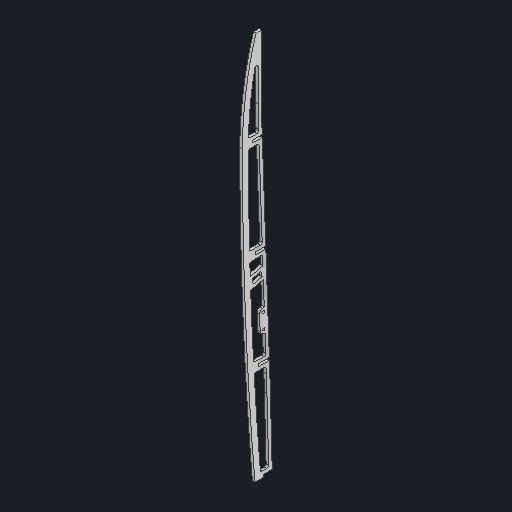
# Autodesk Inventor part: stringer_cowl
Saved by Autodesk Inventor 2023 (Build 270158030, 158C)
## iProperties
Created: 2022-03-23
Part Number: stringer_cowl
Material: Generic
Document SubType Name: Modeling
Designer: kardo
Density: 1 g/cm^3
Appearance: Default
Mass: 17.0204 g
Surface Area: 170.958 cm^2
Volume: 17.0204 cm^3
Author: kardo
Autodesk Inventor part; units mm, degrees
ref_plane "YZ Plane" through (0, 0, 0) normal (1, 0, 0) x (0, 1, 0)
ref_plane "XZ Plane" through (0, 0, 0) normal (0, 1, 0) x (-1, 0, 0)
ref_plane "XY Plane" through (0, 0, 0) normal (0, 0, 1) x (1, 0, 0)
derived "parameters_frame.ipt"
derived "surface_body.ipt"
sketch "sk_rail_top_cowl" plane through (54.6, 0, 0) normal (1, 0, 0) x (0, 1, 0)
  spline S0 degree 2 poles (-345, 39.712) (-172.656, 54.3934) (0, 54.4) knots 0 0 0 1 1 1
  spline S1 degree 3 poles (0, 54.4) (37.026, 54.4) (80.784, 47.9917) (112.2, 37.536) knots 1 1 1 1 2 2 2 2
  point P0 (0, 0)
sketch "sk_rail_bottom_standoff" plane through (34.32, 0, 0) normal (1, 0, 0) x (0, 1, 0)
  line L0 (-345, 16.32) -> (-262.2001, 18.586)
  arc A0 (-262.2001, 18.586) -> (-241.5001, 19.2432) centre (-326.8578, 2381.2399) ccw
  line L1 (36.465, 28.832) -> (112.2, 28.832)
  arc A1 (36.465, 28.832) -> (11.22, 28.376) centre (36.465, -670.197) ccw
  line L2 (-241.5001, 19.2432) -> (11.22, 28.376)
  line L3 (-465, 0) -> (375, 0) construction
  line L4 (11.22, 28.376) -> (11.22, 0) construction
  line L5 (-241.5001, 19.2432) -> (-241.5001, 0) construction
  point P0 (0, 0)
  point P1 (-241.5001, 19.1524)
  point P2 (11.22, 28.832)
ref_plane "plane_middle" through (0, 0, 0) normal (0, 1, 0) x (-1, 0, 0)
ref_plane "plane_rear" through (0, -345, 0) normal (0, 1, 0) x (-1, 0, 0)
ref_plane "plane_cowl_right" through (54.6, 0, 0) normal (1, 0, 0) x (0, 1, 0)
ref_plane "plane_nose" through (0, 112.2, 0) normal (0, 1, 0) x (-1, 0, 0)
ref_plane "plane_tail_1" through (0, -114.9999, 0) normal (0, 1, 0) x (-1, 0, 0)
ref_plane "plane_tail_2" through (0, -230.0001, 0) normal (0, 1, 0) x (-1, 0, 0)
derived "stencil_frame.ipt"
sketch "sk_cowl_joint_locations" plane through (54.6, 0, 0) normal (1, 0, 0) x (0, 1, 0)
  line L0 (-345, 16.32) -> (-262.2001, 18.586) construction
  arc A0 (-262.2001, 18.586) -> (-241.5001, 19.2432) centre (-326.8578, 2381.2399) ccw construction
  line L1 (-241.5001, 19.2432) -> (11.22, 28.376) construction
  arc A1 (36.465, 28.832) -> (11.22, 28.376) centre (36.465, -670.197) ccw construction
  line L2 (36.465, 28.832) -> (112.2, 28.832) construction
  line L3 (94.8, 29.632) -> (36.465, 29.632) construction
  arc A2 (36.465, 29.632) -> (11.1911, 29.1755) centre (36.465, -670.197) ccw construction
  line L4 (11.1911, 29.1755) -> (-241.529, 20.0427) construction
  arc A3 (-262.222, 19.3857) -> (-241.529, 20.0427) centre (-326.8578, 2381.2399) ccw construction
  line L5 (-262.222, 19.3857) -> (-345, 17.1203) construction
  line L6 (-230.0001, 3089.1136) -> (-230.0001, -1866.0023) construction
  line L7 (-114.9999, 3089.1136) -> (-114.9999, -1866.0023) construction
  line L8 (-345, 3089.1136) -> (-345, -1866.0023) construction
  line L9 (0, 3089.1136) -> (0, -1866.0023) construction
  line L10 (-230.0001, 44.8681) -> (-230.0001, 20.4593) construction
  line L11 (-114.9999, 49.7658) -> (-114.9999, 24.6152) construction
  line L12 (-345, 17.1203) -> (-345, 17.1203)
  line L13 (-345, 17.1203) -> (-345, 36.7228) construction
  line L14 (-850.7464, 3011.9134) -> (325.2296, -1886.3794) construction
  line L15 (-344.7454, 36.7228) -> (-345, 39.712) construction
  spline S0 degree 2 poles (-345, 39.712) (-172.656, 54.3934) (0, 54.4) knots 0 0 0 1 1 1
  spline S1 degree 3 poles (0, 54.4) (37.026, 54.4) (80.784, 47.9917) (112.2, 37.536) knots 1 1 1 1 2 2 2 2
  line L16 (0, 51.4) -> (0, 28.7711) construction
  spline S2 degree 3 poles (111.2526, 34.6895) (106.0906, 36.4075) (96.4401, 39.2282) (84.5011, 42.0313) (75.2591, 43.9395) (68.9709, 45.1125) (60.9945, 46.449) (54.5373, 47.4124) (46.413, 48.4791) (39.8882, 49.2203) (31.7426, 50.0013) (25.2514, 50.5076) (17.2112, 50.9875) (9.2661, 51.3118) (3.0567, 51.4) (0, 51.4) knots 1 1 1 1 1.166667 1.291667 1.333333 1.416667 1.458333 1.541667 1.583333 1.666667 1.708333 1.791667 1.833333 1.916667 2 2 2 2
  spline S3 degree 3 poles (0, 51.4) (-19.1698, 51.3993) (-52.712, 51.1604) (-91.0357, 50.4121) (-119.7742, 49.6473) (-138.931, 49.0355) (-162.8744, 48.1436) (-182.0269, 47.3282) (-205.9648, 46.1816) (-225.113, 45.1626) (-249.0455, 43.7615) (-268.1894, 42.5387) (-292.1166, 40.883) (-316.041, 39.1) (-335.1777, 37.5379) (-344.7454, 36.7228) knots 0 0 0 0 0.166667 0.291667 0.333333 0.416667 0.458333 0.541666 0.583333 0.666666 0.708333 0.791666 0.833333 0.916666 1 1 1 1
  line L17 (-144.5331, 44.6212) -> (-139.5174, 23.7292) construction
  line L18 (-134.9371, 30.3529) -> (-140.7713, 28.9522) construction
  line L19 (-137.4449, 40.7989) -> (-143.2792, 39.3982) construction
  line L20 (-144.5331, 44.6212) -> (-138.6989, 46.0219) construction
  line L21 (-139.5174, 23.7292) -> (-133.6831, 25.1299) construction
  line L22 (-138.6989, 46.0219) -> (-138.9044, 52.0184) construction
  point P0 (0, 0)
  point P1 (-345, 26.9216)
  point P2 (-230.0001, 32.6637)
  point P3 (-114.9999, 37.1905)
  point P4 (0, 40.0855)
  point P5 (-850.7464, 3011.9134)
  point P6 (325.2296, -1886.3794)
  point P7 (-85.2629, 50.788)
  point P8 (0, 40.0855)
sketch "sk_servo_mount" plane through (-54.6, 0, 0) normal (1, 0, 0) x (0, 1, 0)
  line L0 (-241.5001, 19.2432) -> (11.22, 28.376) construction
  line L1 (-345, 3089.1136) -> (-345, -1866.0023) construction
  line L2 (0, 3089.1136) -> (0, -1866.0023) construction
  line L3 (-195.0702, 20.9211) -> (-195.2941, 27.117) construction
  line L4 (-195.2941, 27.117) -> (-177.3059, 27.7671) construction
  line L5 (-177.3059, 27.7671) -> (-177.082, 21.5711) construction
  point P0 (0, 0)
  point P1 (-186.3, 27.4421)
sketch "sk_base" plane through (54.6, 0, 0) normal (1, 0, 0) x (0, 1, 0)
  line L0 (-345, 16.32) -> (-262.2001, 18.586) construction
  arc A0 (-262.2001, 18.586) -> (-241.5001, 19.2432) centre (-326.8578, 2381.2399) ccw construction
  line L1 (-241.5001, 19.2432) -> (11.22, 28.376) construction
  arc A1 (36.465, 28.832) -> (11.22, 28.376) centre (36.465, -670.197) ccw construction
  line L2 (36.465, 28.832) -> (112.2, 28.832) construction
  spline S0 degree 3 poles (0, 54.4) (37.026, 54.4) (80.784, 47.9917) (112.2, 37.536) knots 1 1 1 1 2 2 2 2 construction
  spline S1 degree 2 poles (-345, 39.712) (-172.656, 54.3934) (0, 54.4) knots 0 0 0 1 1 1 construction
  line L3 (-345, 2991.5273) -> (-345, -1280.4843) projected
  line L4 (112.2, 2991.5273) -> (112.2, -1280.4843) construction
  line L5 (109.2, 29.632) -> (36.465, 29.632)
  arc A2 (36.465, 29.632) -> (11.1911, 29.1755) centre (36.465, -670.197) ccw
  line L6 (11.1911, 29.1755) -> (-241.529, 20.0427)
  arc A3 (-262.222, 19.3857) -> (-241.529, 20.0427) centre (-326.8578, 2381.2399) ccw
  line L7 (-262.222, 19.3857) -> (-345.0219, 17.1197)
  line L8 (109.2, 36.0963) -> (109.2, 29.632)
  line L9 (-345, 39.712) -> (-344.8048, 37.4203) construction
  line L10 (-344.8048, 37.4203) -> (-345, 37.4037)
  spline S2 degree 4 poles (-344.8048, 37.4203) (-258.811, 44.7458) (-172.6105, 49.6475) (-86.3051, 52.0967) (0.0001, 52.1) knots 0 0 0 0 0 1 1 1 1 1
  spline S3 degree 5 poles (0, 52.1) (11.6181, 52.0997) (23.2348, 51.5721) (34.8234, 50.6426) (56.8455, 48.1371) (78.652, 44.1758) (88.951, 41.9371) (99.1691, 39.3116) (109.1999, 36.0962) knots 0 0 0 0 0 0 0.524477 0.524477 0.524477 1 1 1 1 1 1
  point P0 (0, 0)
  point P1 (-345, 17.1203)
  dimension "d3" = 2.3
  dimension "d2" = 0.8
  dimension "d4" = 3
  constraints: 12 end point, 4 point on circle, 2 centre point, 1 parallel, 1 perpendicular, 1 point on line, 12 other
  measures "d2" distance between parallel lines of L1 L6
  measures "d4" distance between parallel lines of L4 L8
extrude "thicken" add sketch "sk_base" along normal blind 3
sketch "sk_cut_weight" plane through (54.6, 0, 0) normal (1, 0, 0) x (0, 1, 0)
  spline S0 degree 3 poles (-344.8048, 37.4203) (-335.2355, 38.2355) (-316.0955, 39.7979) (-292.1669, 41.5812) (-268.2357, 43.2372) (-249.0885, 44.4601) (-225.1518, 45.8615) (-206.0003, 46.8807) (-182.0583, 48.0275) (-162.9025, 48.843) (-138.955, 49.7351) (-119.7948, 50.347) (-91.0514, 51.1119) (-52.721, 51.8603) (-19.1731, 52.0993) (0, 52.1) knots 0 0 0 0 0.083333 0.166667 0.208333 0.291667 0.333333 0.416667 0.458333 0.541667 0.583333 0.666667 0.708333 0.833333 1 1 1 1 construction
  line L0 (-262.222, 19.3857) -> (-345.0219, 17.1197) construction
  line L1 (109.2, 36.0963) -> (109.2, 29.632) construction
  line L2 (-114.9999, 2991.5273) -> (-114.9999, -1280.4843) construction
  line L3 (-230.0001, 2991.5273) -> (-230.0001, -1280.4843) construction
  line L4 (-345, 2991.5273) -> (-345, -1280.4843) construction
  line L5 (0, 2991.5273) -> (0, -1280.4843) construction
  line L6 (11.1911, 29.1755) -> (-241.529, 20.0427) construction
  arc A0 (-262.222, 19.3857) -> (-241.529, 20.0427) centre (-326.8578, 2381.2399) ccw construction
  line L7 (109.2, 29.632) -> (36.465, 29.632) construction
  arc A1 (36.465, 29.632) -> (11.1911, 29.1755) centre (36.465, -670.197) ccw construction
  spline S1 degree 3 poles (0, 52.1) (2.9894, 52.1) (9.0592, 52.0158) (16.8211, 51.7063) (24.675, 51.2481) (31.016, 50.7645) (38.9753, 50.0185) (45.3538, 49.3103) (53.3014, 48.2907) (59.6236, 47.3694) (67.4424, 46.0908) (73.6147, 44.9683) (81.1874, 43.4456) (87.1158, 42.1337) (94.3247, 40.3821) (101.3124, 38.5213) (106.6243, 36.922) (109.2, 36.0963) knots 1 1 1 1 1.081321 1.162641 1.203301 1.284622 1.325282 1.406602 1.447263 1.528583 1.569243 1.650564 1.691224 1.772544 1.813204 1.894525 1.975845 1.975845 1.975845 1.975845 construction
  line L8 (-342, 17.1197) -> (-342, 52.1) construction
  line L9 (-227.0001, 52.1) -> (-227.0001, 17.1197) construction
  line L10 (-111.9999, 52.1) -> (-111.9999, 17.1197) construction
  line L11 (3, 52.1) -> (3, 17.1197) construction
  line L12 (-338, 30.9698) -> (-338, 21.3134)
  line L13 (-234.0001, 24.3174) -> (-234.0001, 38.3285)
  line L14 (-223.0001, 38.9501) -> (-223.0001, 24.7149)
  line L15 (-107.9999, 43.6563) -> (-107.9999, 28.8708)
  line L16 (-4, 32.6291) -> (-4, 45.0979)
  line L17 (7, 45.0237) -> (7, 33.0266)
  line L18 (92.3656, 33.632) -> (36.465, 33.632)
  arc A2 (36.465, 33.632) -> (11.0467, 33.1729) centre (36.465, -670.197) ccw
  line L19 (11.0467, 33.1729) -> (-241.6735, 24.0401)
  arc A3 (-262.3314, 23.3842) -> (-241.6735, 24.0401) centre (-326.8578, 2381.2399) ccw
  line L20 (-262.3314, 23.3842) -> (-342, 21.2039)
  line L21 (-118.9999, 43.3476) -> (-118.9999, 28.4733)
  spline S2 degree 5 poles (92.3656, 33.6321) (85.0708, 35.4926) (77.7159, 37.1178) (70.3234, 38.553) (51.9201, 41.6659) (33.3653, 43.7323) (22.2612, 44.6046) (11.1313, 45.0997) (0, 45.1) knots 0 0 0 0 0 0 0.40346 0.40346 0.40346 1 1 1 1 1 1
  spline S3 degree 4 poles (0.0003, 45.1) (-85.6016, 45.0967) (-171.2037, 42.6831) (-256.703, 37.8526) (-342, 30.6333) knots 0 0 0 0 0 1 1 1 1 1
  point P0 (0, 0)
  dimension "d51" = 7
  dimension "d18" = 3
  dimension "d19" = 3
  dimension "d20" = 3
  dimension "d21" = 3
  dimension "d22" = 4
  dimension "d23" = 4
  dimension "d26" = 4
  dimension "d27" = 4
  dimension "d28" = 4
  dimension "d29" = 4
  dimension "d30" = 4
  dimension "d52" = 4
  constraints: 28 end point, 11 parallel, 9 point on line, 8 horizontal alignment, 4 point on circle, 2 centre point, 17 other
  measures "d18" distance between parallel lines of L3 L9
  measures "d19" distance between parallel lines of L10 L2
  measures "d20" distance between parallel lines of L11 L5
  measures "d21" distance between parallel lines of L8 L4
  measures "d22" distance between parallel lines of L8 L12
  measures "d23" distance between parallel lines of L13 L3
  measures "d26" distance between parallel lines of L9 L14
  measures "d27" distance between parallel lines of L10 L15
  measures "d28" distance between parallel lines of L16 L5
  measures "d29" distance between parallel lines of L11 L17
  measures "d30" distance between parallel lines of L21 L2
  measures "d52" distance between parallel lines of L7 L18
extrude "cut_weight" cut sketch "sk_cut_weight" along normal through all both and the other way through all contours S3 L13 L19 A3 L20 L12 | S3 L21 L19 L14 | S3 L16 L19 L15 | L17 S2 L18 A2 L19
fillet "rounding" radius 2 15 edges at (56.1, -234.0001, 24.3174) (56.1, -118.9999, 28.4733) (56.1, -4, 32.6291) (56.1, 7, 33.0266) (56.1, -107.9999, 28.8708) (56.1, -223.0001, 24.7149) (56.1, -338, 21.3134) (56.1, -338, 30.9698) (56.1, -223.0001, 38.9501) (56.1, -107.9999, 43.6563) (56.1, 7, 45.0237) (56.1, -4, 45.0979) (56.1, -118.9999, 43.3476) (56.1, -234.0001, 38.3285) (56.1, 92.3656, 33.632)
sketch "sk_joint_motor_mount" plane through (54.6, 0, 0) normal (1, 0, 0) x (0, 1, 0)
  spline S0 degree 3 poles (-344.8048, 37.4203) (-335.2355, 38.2355) (-316.0955, 39.7979) (-292.1669, 41.5812) (-268.2357, 43.2372) (-249.0885, 44.4601) (-225.1518, 45.8615) (-206.0003, 46.8807) (-182.0583, 48.0275) (-162.9025, 48.843) (-138.955, 49.7351) (-119.7948, 50.347) (-91.0514, 51.1119) (-52.721, 51.8603) (-19.1731, 52.0993) (0, 52.1) knots 0 0 0 0 0.083333 0.166667 0.208333 0.291667 0.333333 0.416667 0.458333 0.541667 0.583333 0.666667 0.708333 0.833333 1 1 1 1 projected
  line L0 (11.1911, 29.1755) -> (-241.529, 20.0427) projected
  line L1 (-137.4449, 40.7989) -> (-134.9371, 30.3529) construction
  line L2 (-137.4449, 40.7989) -> (-143.2792, 39.3982) construction
  line L3 (-143.2792, 39.3982) -> (-140.7713, 28.9522) construction
  line L4 (-140.7713, 28.9522) -> (-134.9371, 30.3529) construction
  line L5 (-149.7772, 49.3297) -> (-143.5956, 23.5818)
  line L6 (-135.5, 49.8323) -> (-129.3217, 24.0976)
  point P0 (0, 0)
  dimension "d33" = 6
  dimension "d34" = 4
  dimension "d35" = 4
  constraints: 12 end point, 3 parallel, 2 coincident, 2 perpendicular, 2 point on line, 2 other
  measures "d33" distance between parallel lines of L1 L3
  measures "d34" distance between parallel lines of L3 L5
  measures "d35" distance between parallel lines of L1 L6
extrude "joint_motor_mount" add sketch "sk_joint_motor_mount" along normal blind 3
sketch "sk_joint_servo" plane through (54.6, 0, 0) normal (1, 0, 0) x (0, 1, 0)
  line L0 (11.1911, 29.1755) -> (-241.529, 20.0427) projected
  line L1 (-171.8973, 22.559) -> (-173.1987, 28.6453)
  arc A0 (-173.1987, 28.6453) -> (-177.4576, 31.9644) centre (-177.3059, 27.7671) ccw
  line L2 (-177.4576, 31.9644) -> (-195.4458, 31.3143)
  arc A1 (-195.4458, 31.3143) -> (-199.454, 27.6965) centre (-195.2941, 27.117) ccw
  line L3 (-199.454, 27.6965) -> (-200.3127, 21.5322)
  point P0 (0, 0)
  dimension "d39" = 80
  dimension "d40" = 80
  dimension "d41" = 4.2
  constraints: 6 end point, 4 point on circle, 4 tangent, 2 centre point, 2 coincident, 2 point on line, 1 equal radius
  measures "d39" angle of L1 L0
  measures "d40" angle of L0 L3
  measures "d41" radius of A0
extrude "joint_servo" add sketch "sk_joint_servo" along normal blind 3
hole "drill_joint_servo" at (54.6, -195.2941, 27.117) at (54.6, -177.3059, 27.7671) direction (1, 0, 0) diameter 3 end through all
sketch "sk_cowl_joint_cuts" plane through (54.6, 0, 0) normal (1, 0, 0) x (0, 1, 0)
  line L0 (-230.0001, 2991.5273) -> (-230.0001, -1280.4843) projected
  line L1 (-114.9999, 2991.5273) -> (-114.9999, -1280.4843) projected
  line L2 (0, 2991.5273) -> (0, -1280.4843) projected
  line L3 (-345, 2991.5273) -> (-345, -1280.4843) projected
  line L4 (-114.9999, -12.8095) -> (-111.9999, -12.8095)
  line L5 (-111.9999, -12.8095) -> (-111.9999, 37.1905)
  line L6 (-111.9999, 37.1905) -> (-114.9999, 37.1905)
  line L7 (0, -9.9145) -> (3, -9.9145)
  line L8 (3, -9.9145) -> (3, 40.0855)
  line L9 (3, 40.0855) -> (0, 40.0855)
  line L10 (-230.0001, 32.6637) -> (-227.0001, 32.6637)
  line L11 (-227.0001, 32.6637) -> (-227.0001, -17.3363)
  line L12 (-227.0001, -17.3363) -> (-230.0001, -17.3363)
  line L13 (-345, 26.9216) -> (-342, 26.9216)
  line L14 (-342, 26.9216) -> (-342, -23.0784)
  line L15 (-342, -23.0784) -> (-345, -23.0784)
  line L16 (-134.9371, 30.3529) -> (-137.4449, 40.7989)
  line L17 (-137.4449, 40.7989) -> (-143.2792, 39.3982)
  line L18 (-143.2792, 39.3982) -> (-140.7713, 28.9522)
  line L19 (-140.7713, 28.9522) -> (-134.9371, 30.3529)
  point P0 (0, 0)
  dimension "d8" = 3
  dimension "d15" = 50
  dimension "d16" = 6
  constraints: 33 end point, 11 parallel, 10 perpendicular, 4 point on line
  measures "d8" distance of L8.end L9.end
  measures "d15" distance of L7.end L8.end
  measures "d16" distance of L16.end L17.end
extrude "cut_joints" cut sketch "sk_cowl_joint_cuts" along normal through all
equation "\"d2\" = shell_thickness"
equation "\"d5\" = bulkhead_thickness"
equation "\"d51\" = bulkhead_inset + cowl_sealing_thickness"
equation "\"d18\" = bulkhead_thickness"
equation "\"d19\" = bulkhead_thickness"
equation "\"d20\" = bulkhead_thickness"
equation "\"d21\" = bulkhead_thickness"
equation "\"d22\" = bulkhead_inset"
equation "\"d23\" = bulkhead_inset"
equation "\"d26\" = bulkhead_inset"
equation "\"d27\" = bulkhead_inset"
equation "\"d28\" = bulkhead_inset"
equation "\"d29\" = bulkhead_inset"
equation "\"d30\" = bulkhead_inset"
equation "\"d38\" = 0.5 * bulkhead_inset"
equation "\"d33\" = 2 * bulkhead_thickness"
equation "\"d34\" = bulkhead_inset"
equation "\"d35\" = bulkhead_inset"
equation "\"d36\" = bulkhead_thickness"
equation "\"d41\" = 1.4 * drill_servo_mount_diam"
equation "\"d42\" = bulkhead_thickness"
equation "\"d44\" = drill_servo_mount_diam"
equation "\"d8\" = bulkhead_thickness"
equation "\"d16\" = 2 * bulkhead_thickness"
equation "\"shell_thickness\" = 0.8"
equation "\"bulkhead_thickness\" = 3"
equation "\"bulkhead_inset\" = 4"
equation "\"cowl_sealing_thickness\" = 3"
equation "\"drill_servo_mount_diam\" = 3"
body "Solid1"
